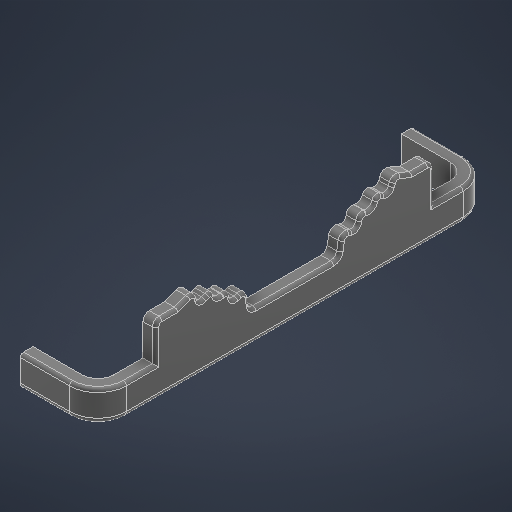
# Autodesk Inventor part: Bumper Delantero
Saved by Autodesk Inventor 2026.2 (Build 302298000, 298)
## iProperties
Created: 2026-02-05
Part Number: Bumper Delantero
Material: Generic
Document SubType Name: Modeling
Designer: 06aar
Density: 1 g/cm^3
Appearance: Smooth - Black
Author: 06aar
Autodesk Inventor part; units mm, degrees
ref_plane "YZ Plane" through (0, 0, 0) normal (1, 0, 0) x (0, 1, 0)
ref_plane "XZ Plane" through (0, 0, 0) normal (0, 1, 0) x (-1, 0, 0)
ref_plane "XY Plane" through (0, 0, 0) normal (0, 0, 1) x (1, 0, 0)
sketch "Sketch1" plane through (0, 0, 0) normal (0, 1, 0) x (-1, 0, 0)
  line L0 (0, 0) -> (4, 0)
  line L1 (4, 0) -> (4, 62.2232)
  line L2 (4, 62.2232) -> (0, 62.2232)
  line L3 (0, 62.2232) -> (0, 0)
  line L4 (4, 62.2232) -> (24.5, 62.2232)
  line L5 (24.5, 62.2232) -> (24.5, 58.2232)
  line L6 (24.5, 58.2232) -> (4, 58.2232)
  line L7 (4, 58.2232) -> (4, 62.2232)
  circle A0 centre (10, 33.2232) radius 1.55
  circle A1 centre (10, 33.2232) radius 3.55
  line L8 (4, 39.1116) -> (11.184, 36.57)
  line L9 (4, 23.1116) -> (12.3635, 30.5744)
  line L10 (10, 33.2232) -> (4, 31.1116)
  point P0 (4, 58.2232)
  dimension "d0" = 62.2232
  dimension "d1" = 4
  dimension "d2" = 20.5
  dimension "d3" = 4
  dimension "d4" = 6
  dimension "d5" = 3.1
  dimension "d6" = 25
  dimension "d7" = 2
  dimension "d10" = 8
  dimension "d11" = 8
  constraints: 22 end point, 4 parallel, 2 centre point, 2 horizontal, 2 perpendicular, 2 point on circle, 2 point on line, 2 tangent, 1 coincident, 1 midpoint
  measures "d0" distance of L2.end L0.start
  measures "d1" distance between parallel lines of L3 L1
  measures "d2" distance of L1.end L4.end
  measures "d3" distance of L4.end L5.end
  measures "d4" distance from line of L1 A0.centre
  measures "d5" diameter of A0
  measures "d6" distance from line of L6 A0.centre
  measures "d7" radial gap between concentric circles of A0 A1
  measures "d10" distance of L10.end L8.start
  measures "d11" distance of L9.start L10.end
extrude "Extrusion1" add sketch "Sketch1" along normal blind 10 contours L3 L2 L1 L0 | L4 L5 L6 L1
extrude "Extrusion2" add sketch "Sketch1" along normal blind 3 contours L1 L10 A1 L9 | L1 L8 A1 L10 | A1
fillet "Fillet1" radius 5 1 edges at (-4, 5, 58.2232)
fillet "Fillet2" radius 9 1 edges at (0, 5, 62.2232)
fillet "Fillet3" radius 2 3 edges at (0, 0, 26.6116) (-16.75, 0, 62.2232) (-2.636, 0, 59.5872)
fillet "Fillet5" radius 1 2 edges at (-4, 1.5, 23.1116) (-4, 1.5, 39.1116)
sketch "Sketch3" plane through (0, 10, 53.2232) normal (1, 0, 0) x (0, 0, -1)
  line L0 (0, 0) -> (53.2232, 0) projected
  line L1 (39.2232, 0) -> (9.2232, 0)
  line L2 (9.2232, 0) -> (9.2232, 12)
  line L3 (9.2232, 12) -> (39.2232, 12)
  line L4 (39.2232, 12) -> (39.2232, 0)
  line L5 (53.2232, -8) -> (53.2232, 0) projected
  arc A0 (39.2232, 0) -> (9.2232, 12) centre (9.2232, -31.5) ccw
  line L6 (16.146, 12) -> (21.6375, 14.2875)
  line L7 (21.6375, 14.2875) -> (23.225, 9.685)
  line L8 (23.225, 9.685) -> (27.7169, 12)
  line L9 (27.9158, 7.779) -> (27.7169, 12)
  line L10 (27.9158, 7.779) -> (32.9779, 9.525)
  line L11 (32.9779, 9.525) -> (32.9779, 4.9413)
  line L12 (32.9779, 4.9413) -> (38.1465, 6.724)
  line L13 (38.1465, 6.724) -> (39.2232, 0)
  point P0 (53.2232, -10)
  point P1 (33.4403, 4.6356)
  point P2 (38.4497, 0.719)
  point P3 (9.2232, 0)
  dimension "d29" = 14
  dimension "d30" = 12
  dimension "d31" = 30
  constraints: 24 end point, 7 point on circle, 3 parallel, 3 point on line, 2 perpendicular, 1 centre point, 1 horizontal, 1 tangent, 1 vertical
  measures "d29" distance between parallel lines of L5 L4
  measures "d30" distance between parallel lines of L0 L3
  measures "d31" distance between parallel lines of L4 L2
extrude "Extrusion4" add sketch "Sketch3" against normal blind 4 contours L2 A0 L0 | A0 L12 L13 | L3 L7 A0 | A0 L10 L11 | L6 L7 L3 | L8 L9 A0
fillet "Fillet16" radius 2 4 edges at (-2, 24.2875, 31.5857) (-2, 16.724, 15.0767) (-2, 10, 14) (-2, 17.779, 25.3075)
fillet "Fillet17" radius 1.5 3 edges at (-2, 19.685, 29.9982) (-2, 22, 25.5063) (-2, 14.9413, 20.2454)
fillet "Fillet18" radius 1.8 1 edges at (-2, 19.525, 20.2454)
fillet "Fillet19" radius 2 1 edges at (-2, 22, 44)
ref_plane "Work Plane2" through (-2, 10, 0) normal (0, 0, -1) x (-1, 0, 0)
mirror "Mirror1" about plane through (-2, 10, 0) normal (0, 0, -1)
fillet "Fillet20" radius 1 3 edges at (-16.75, 10, 62.2232) (0, 10, 48.6116) (-2.636, 10, 59.5872)
fillet "Fillet21" radius 1 27 edges at (0, 10, 0) (0, 10.4781, -13.5924) (0, 13.0285, -14.4849) (0, 15.7726, -15.647) (0, 15.7876, -17.7918) (0, 15.818, -19.6077) (0, 18.473, -21.0102) (0, 18.7746, -24.3745) (0, 21.0086, -26.2093) (0, 20.7246, -27.981) (0, 20.4199, -29.7035) (0, 21.7988, -30.7274) (0, 23.4471, -31.963) (0, 22.7344, -35.3142) (0, 10.4781, 13.5924) (0, 13.0285, 14.4849) (0, 15.7726, 15.647) (0, 15.7876, 17.7918) (0, 15.818, 19.6077) (0, 18.473, 21.0102) (0, 18.7746, 24.3745) (0, 21.0086, 26.2093) (0, 20.7246, 27.981) (0, 20.4199, 29.7035) (0, 21.7988, 30.7274) (0, 23.4471, 31.963) (0, 22.7344, 35.3142)
fillet "Fillet22" radius 1 12 edges at (0, 21.4142, 43.4142) (0, 22, 39.5386) (0, 22, 35.777) (0, 9.5, 44) (0, 15, 44) (0, 21.4142, -43.4142) (0, 22, -35.777) (0, 22, -39.5386) (0, 15, -44) (-2.636, 10, -59.5872) (-16.75, 10, -62.2232) (0, 10, -48.6116)
body "Solid1"
